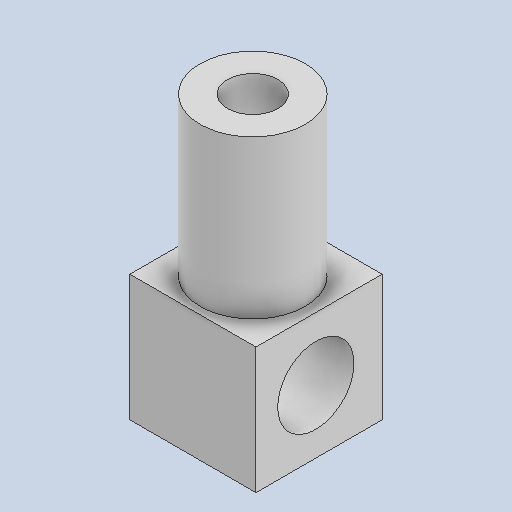
# Autodesk Inventor part: corrector
Saved by Autodesk Inventor 2025 (Build 290162000, 162)
## iProperties
Created: 2025-07-16
Part Number: corrector
Material: Generic
Document SubType Name: Modeling
Designer: Pravoslav
Density: 1 g/cm^3
Appearance: Default
Author: Pravoslav
Autodesk Inventor part; units mm, degrees
ref_plane "YZ Plane" through (0, 0, 0) normal (1, 0, 0) x (0, 1, 0)
ref_plane "XZ Plane" through (0, 0, 0) normal (0, 1, 0) x (-1, 0, 0)
ref_plane "XY Plane" through (0, 0, 0) normal (0, 0, 1) x (1, 0, 0)
sketch "Sketch1" plane through (0, 0, 0) normal (1, 0, 0) x (0, 1, 0)
  line L0 (6, 5.6915) -> (-6, 5.6915)
  line L1 (-6, 5.6915) -> (-6, -6.3085)
  line L2 (-6, -6.3085) -> (6, -6.3085)
  line L3 (6, -6.3085) -> (6, 5.6915)
  line L4 (6, 5.6915) -> (-6, -6.3085) construction
  line L5 (-6, 5.6915) -> (6, -6.3085) construction
  point P0 (0, 0)
  point P1 (0, -0.3085)
  dimension "d0" = 12
  dimension "d1" = 12
  constraints: 12 end point, 2 midpoint, 2 parallel, 1 horizontal, 1 perpendicular
  measures "d0" distance of L2.end L1.end
  measures "d1" distance of L1.end L0.end
extrude "Extrusion1" add sketch "Sketch1" along normal mid plane 12
sketch "Sketch2" plane through (6, 0, 0) normal (1, 0, 0) x (0, 0, -1)
  circle A0 centre (0, 0) radius 3.625
  dimension "d4" = 7.25
  constraints: 1 centre point, 1 coincident
  measures "d4" diameter of A0
extrude "Extrusion2" cut sketch "Sketch2" against normal through all
sketch "Sketch3" plane through (-6, 6, 5.6915) normal (0, 1, 0) x (1, 0, 0)
  circle A0 centre (6, 5.6915) radius 2.4
  dimension "d7" = 4.8
  constraints: 1 centre point, 1 coincident
  measures "d7" diameter of A0
extrude "Extrusion3" cut sketch "Sketch3" against normal up to surface round surface about axis through (6, 0, 0) along (-1, 0, 0) radius 3.625 far side no
sketch "Sketch4" plane through (-6, 6, 5.6915) normal (0, 1, 0) x (1, 0, 0)
  circle A0 centre (6, 5.6915) radius 5
  circle A1 centre (6, 5.6915) radius 2.4
  dimension "d10" = 10
  constraints: 2 centre point, 2 coincident
  measures "d10" diameter of A0
extrude "Extrusion4" add sketch "Sketch4" along normal blind 15
body "Solid1"
